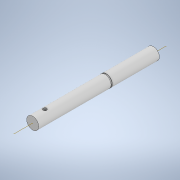
# Autodesk Inventor part: Shaft_piston
Saved by Autodesk Inventor 2022 (Build 260153000, 153)
## iProperties
Created: 2022-04-21
Part Number: Shaft_piston
Material: Generic
Document SubType Name: Sheet Metal
Designer: Malaika Din Hashmi
Density: 1 g/cm^3
Sheet Metal Rule: Default
Appearance: Default
Author: Malaika Din Hashmi
Autodesk Inventor part; units mm, degrees
ref_plane "YZ Plane" through (0, 0, 0) normal (1, 0, 0) x (0, 1, 0)
ref_plane "XZ Plane" through (0, 0, 0) normal (0, 1, 0) x (-1, 0, 0)
ref_plane "XY Plane" through (0, 0, 0) normal (0, 0, 1) x (1, 0, 0)
sketch "Sketch3" plane through (0, 0, 0) normal (0, 0, 1) x (1, 0, 0)
  circle A0 centre (0, 0) radius 5
  dimension "d0" = 10
  constraints: 1 centre point, 1 coincident
  measures "d0" diameter of A0
extrude "Extrusion1" add sketch "Sketch3" against normal blind 100
sketch "Sketch4" plane through (0, 0, 0) normal (0, 1, 0) x (-1, 0, 0)
  circle A0 centre (0, -10) radius 1.5
  line L0 (5, 0) -> (-5, 0) projected
  point P0 (0, 0)
  dimension "d3" = 3
  dimension "d11" = 10
  constraints: 1 centre point
  measures "d3" diameter of A0
  measures "d11" distance from line of A0.centre L0
hole "Hole1" at (0, 0, -10) direction (0, -1, 0) diameter 3 end through all both
sketch "Sketch14" plane through (0, 0, 0) normal (0, 1, 0) x (-1, 0, 0)
  line L0 (-5, 0) -> (-5, -100) projected
  line L1 (-5, -61) -> (-4.6, -61)
  line L2 (-4.6, -61) -> (-4.6, -60)
  line L3 (-4.6, -60) -> (-5, -60)
  line L4 (-5, -60) -> (-5, -61)
  line L5 (5, 0) -> (-5, 0) projected
  line L6 (0, -120) -> (0, 20) projected
  point P0 (0, 0)
  dimension "d22" = 60
  dimension "d23" = 0.4
  dimension "d24" = 1
  constraints: 8 end point, 2 parallel, 1 horizontal, 1 perpendicular, 1 point on line
  measures "d22" distance between parallel lines of L5 L3
  measures "d23" distance of L1.start L1.end
  measures "d24" distance of L1.end L2.end
revolve "Revolution2" cut sketch "Sketch14" angle 360 about axis through (0, 0, 0) along (0, 0, -1)
equation "\"BendRadius\" = Thickness"
equation "\"BendReliefWidth\" = Thickness"
equation "\"BendReliefDepth\" = 0.5 * Thickness"
equation "\"CornerReliefSize\" = 4 * Thickness"
equation "\"MinimumRemnant\" = 2 * Thickness"
equation "\"TransitionRadius\" = BendRadius"
equation "\"JacobiRadiusSize\" = BendRadius"
equation "\"GapSize\" = Thickness"
equation "\"Thickness\" = 3.048"
body "Solid1"
